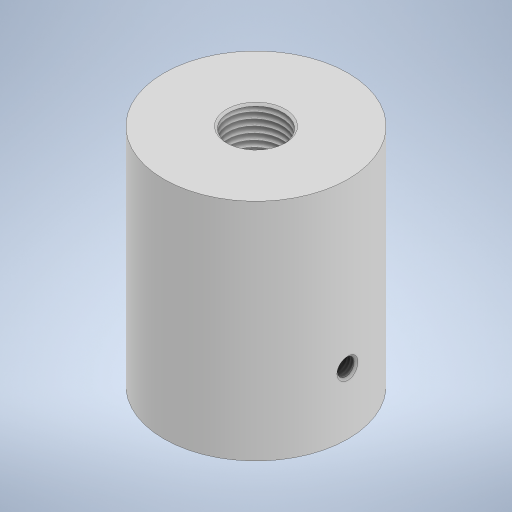
# Autodesk Inventor part: Маховик
Saved by Autodesk Inventor 2023 (Build 270158000, 158)
## iProperties
Created: 2022-05-01
Part Number: Маховик
Material: Типовые
Document SubType Name: Modeling
Designer: User
Density: 1 g/cm^3
Appearance: По умолчанию
Author: User
Autodesk Inventor part; units mm, degrees
ref_plane "YZ Plane" through (0, 0, 0) normal (1, 0, 0) x (0, 1, 0)
ref_plane "XZ Plane" through (0, 0, 0) normal (0, 1, 0) x (-1, 0, 0)
ref_plane "XY Plane" through (0, 0, 0) normal (0, 0, 1) x (1, 0, 0)
sketch "Эскиз1" plane through (0, 0, 0) normal (0, 1, 0) x (-1, 0, 0)
  circle A0 centre (0, 0) radius 22.5
  dimension "d0" = 45
  constraints: 1 centre point, 1 coincident
  measures "d0" diameter of A0
extrude "Выдавливание1" add sketch "Эскиз1" along normal blind 55
sketch "Эскиз2" plane through (0, 0, 0) normal (0, -1, 0) x (1, 0, 0)
  circle A0 centre (0, 0) radius 22.5 projected
  point P0 (22.5, 0)
  constraints: 1 horizontal alignment, 1 other
ref_plane "РабПлоскость1" through (22.5, 0, 0) normal (1, 0, 0) x (0, 1, 0)
sketch "Эскиз3" plane through (22.5, 0, 0) normal (1, 0, 0) x (0, 1, 0)
  line L0 (0, 0) -> (12.5, 0)
  line L1 (12.5, 0) -> (17.5, 0)
  circle A0 centre (15, 0) radius 2.5
  dimension "d3" = 12.5
  dimension "d4" = 5
  constraints: 4 end point, 1 horizontal, 1 horizontal alignment, 1 midpoint, 1 point on line, 2 other
  measures "d3" distance of L0.start L0.end
  measures "d4" distance of L0.end L1.end
hole "Отверстие1" at (22.5, 15, 0) direction (-1, 0, 0) diameter 4.134 depth 14.2 tip angle 118 thread size "M5x0.8" class "6H" standard "ISO Metric profile"
chamfer "Фаска1" distance 0.5 angle 45 3 edges at (22.4049, 14.9998, 2.067) (22.4453, 16.3469, -1.5679) (22.4452, 13.6549, -1.5695)
sketch "Эскиз4" plane through (0, 55, 0) normal (0, 1, 0) x (1, 0, 0)
  point P0 (0, 0)
  point P1 (0, 0)
  constraints: 1 coincident
hole "Отверстие2" at (0, 55, 0) direction (0, -1, 0) diameter 13.3762 depth 20 tip angle 118 thread size "M15x1.5" class "6H" standard "ISO Metric profile"
chamfer "Фаска2" distance 0.5 angle 45 1 edges at (0, 55, -6.6881)
sketch "Эскиз5" plane through (0, 0, 0) normal (0, -1, 0) x (1, 0, 0)
  circle A0 centre (0, 0) radius 8
  dimension "d27" = 16
  constraints: 1 centre point, 1 coincident
  measures "d27" diameter of A0
extrude "Выдавливание2" cut sketch "Эскиз5" against normal blind 4
sketch "Эскиз6" plane through (0, 0, 0) normal (0, -1, 0) x (1, 0, 0)
  circle A0 centre (0, 0) radius 22.5
  circle A1 centre (0, 0) radius 8 projected
  line L0 (8, 0) -> (22.5, 0)
  circle A2 centre (0, 0) radius 15.5
  line L1 (15.5, 15.5) -> (-15.5, 15.5)
  line L2 (-15.5, 15.5) -> (-15.5, -15.5)
  line L3 (-15.5, -15.5) -> (15.5, -15.5)
  line L4 (15.5, -15.5) -> (15.5, 15.5)
  line L5 (-15.5, -15.5) -> (15.5, 15.5)
  line L6 (15.5, -15.5) -> (-15.5, 15.5)
  point P0 (10.9602, 10.9602)
  point P1 (10.9602, -10.9602)
  point P2 (-10.9602, -10.9602)
  point P3 (-10.9602, 10.9602)
  dimension "d30" = 45
  dimension "d31" = 31
  constraints: 14 end point, 4 point on circle, 4 point on line, 2 coincident, 2 horizontal, 2 horizontal alignment, 2 parallel, 2 perpendicular, 1 centre point, 3 other
  measures "d31" diameter of A2
hole "Отверстие3" at (10.9602, 0, 10.9602) at (10.9602, 0, -10.9602) at (-10.9602, 0, -10.9602) at (-10.9602, 0, 10.9602) direction (0, 1, 0) diameter 2.459 depth 8 tip angle 118 thread size "M3x0.5" class "6H" standard "ISO Metric profile"
chamfer "Фаска3" distance 0.5 angle 45 4 edges at (10.9602, 0, 12.1897) (-10.9602, 0, 12.1897) (-10.9602, 0, -9.7307) (10.9602, 0, -9.7307)
